Autodesk Fusion 360 part; units mm, degrees
(part 7 of 7)
  spline S2021 degree 3 poles (-41.0081, 27.0862) (-40.9963, 27.0636) (-41.0844, 27.0271) (-41.1005, 27.0604) knots 0 0 0 0 1 1 1 1
  spline S2022 degree 3 poles (-41.1005, 27.0604) (-41.1284, 27.1281) (-41.1295, 27.1399) (-41.1349, 27.1904) knots 0 0 0 0 1 1 1 1
  spline S2023 degree 3 poles (-38.245, 28.2123) (-38.2557, 28.2779) (-38.1913, 28.3445) (-38.1558, 28.251) knots 0 0 0 0 1 1 1 1
  spline S2024 degree 3 poles (-38.1558, 28.251) (-38.1258, 28.1715) (-38.129, 28.1296) (-38.1182, 28.107) knots 0 0 0 0 1 1 1 1
  spline S2025 degree 3 poles (-38.1182, 28.107) (-38.1064, 28.0845) (-38.1945, 28.049) (-38.2106, 28.0823) knots 0 0 0 0 1 1 1 1
  spline S2026 degree 3 poles (-38.2106, 28.0823) (-38.2386, 28.1489) (-38.2396, 28.1618) (-38.245, 28.2123) knots 0 0 0 0 1 1 1 1
  spline S2027 degree 3 poles (-40.9179, 27.2764) (-40.9318, 27.3473) (-40.8609, 27.4236) (-40.8233, 27.3258) knots 0 0 0 0 1 1 1 1
  spline S2028 degree 3 poles (-40.8233, 27.3258) (-40.789, 27.2398) (-40.7954, 27.199) (-40.7804, 27.1689) knots 0 0 0 0 1 1 1 1
  spline S2029 degree 3 poles (-40.7804, 27.1689) (-40.7664, 27.1388) (-40.8609, 27.098) (-40.8803, 27.1377) knots 0 0 0 0 1 1 1 1
  spline S2030 degree 3 poles (-40.8803, 27.1377) (-40.9082, 27.2033) (-40.9104, 27.2259) (-40.9179, 27.2764) knots 0 0 0 0 1 1 1 1
  spline S2031 degree 3 poles (-38.4889, 28.1468) (-38.5039, 28.2177) (-38.4341, 28.294) (-38.3954, 28.1962) knots 0 0 0 0 1 1 1 1
  spline S2032 degree 3 poles (-38.3954, 28.1962) (-38.361, 28.1103) (-38.3685, 28.0705) (-38.3535, 28.0404) knots 0 0 0 0 1 1 1 1
  spline S2033 degree 3 poles (-38.3535, 28.0404) (-38.3385, 28.0103) (-38.4341, 27.9695) (-38.4523, 28.0082) knots 0 0 0 0 1 1 1 1
  spline S2034 degree 3 poles (-38.4523, 28.0082) (-38.4813, 28.0748) (-38.4824, 28.0963) (-38.4889, 28.1468) knots 0 0 0 0 1 1 1 1
  spline S2035 degree 3 poles (-40.6998, 27.3613) (-40.7181, 27.4386) (-40.6418, 27.5224) (-40.601, 27.4214) knots 0 0 0 0 1 1 1 1
  spline S2036 degree 3 poles (-40.601, 27.4214) (-40.5644, 27.329) (-40.572, 27.2903) (-40.5537, 27.2527) knots 0 0 0 0 1 1 1 1
  spline S2037 degree 3 poles (-40.5537, 27.2527) (-40.5354, 27.2151) (-40.6386, 27.1689) (-40.66, 27.214) knots 0 0 0 0 1 1 1 1
  spline S2038 degree 3 poles (-40.66, 27.214) (-40.6901, 27.2807) (-40.6901, 27.3118) (-40.6998, 27.3613) knots 0 0 0 0 1 1 1 1
  spline S2039 degree 3 poles (-38.737, 28.0307) (-38.7553, 28.107) (-38.679, 28.1919) (-38.6382, 28.0909) knots 0 0 0 0 1 1 1 1
  spline S2040 degree 3 poles (-38.6382, 28.0909) (-38.6006, 27.9985) (-38.6092, 27.9587) (-38.5909, 27.9211) knots 0 0 0 0 1 1 1 1
  spline S2041 degree 3 poles (-38.5909, 27.9211) (-38.5727, 27.8846) (-38.6758, 27.8373) (-38.6973, 27.8824) knots 0 0 0 0 1 1 1 1
  spline S2042 degree 3 poles (-38.6973, 27.8824) (-38.7263, 27.9491) (-38.7274, 27.9802) (-38.737, 28.0307) knots 0 0 0 0 1 1 1 1
  spline S2043 degree 3 poles (-40.4828, 27.4472) (-40.5043, 27.5289) (-40.4216, 27.6224) (-40.3786, 27.5171) knots 0 0 0 0 1 1 1 1
  spline S2044 degree 3 poles (-40.3786, 27.5171) (-40.3388, 27.4193) (-40.3496, 27.3817) (-40.3259, 27.3366) knots 0 0 0 0 1 1 1 1
  spline S2045 degree 3 poles (-40.3259, 27.3366) (-40.3044, 27.2914) (-40.4151, 27.2398) (-40.4398, 27.2903) knots 0 0 0 0 1 1 1 1
  spline S2046 degree 3 poles (-40.4398, 27.2903) (-40.471, 27.357) (-40.471, 27.3967) (-40.4828, 27.4472) knots 0 0 0 0 1 1 1 1
  spline S2047 degree 3 poles (-39.0443, 27.9534) (-39.0658, 28.034) (-38.982, 28.1285) (-38.9401, 28.0232) knots 0 0 0 0 1 1 1 1
  spline S2048 degree 3 poles (-38.9401, 28.0232) (-38.8993, 27.9243) (-38.91, 27.8867) (-38.8874, 27.8416) knots 0 0 0 0 1 1 1 1
  spline S2049 degree 3 poles (-38.8874, 27.8416) (-38.8659, 27.7976) (-38.9777, 27.7449) (-39.0013, 27.7954) knots 0 0 0 0 1 1 1 1
  spline S2050 degree 3 poles (-39.0013, 27.7954) (-39.0314, 27.8631) (-39.0325, 27.9029) (-39.0443, 27.9534) knots 0 0 0 0 1 1 1 1
  spline S2051 degree 3 poles (-39.2119, 28.5068) (-39.2334, 28.5884) (-39.1517, 28.6819) (-39.1087, 28.5777) knots 0 0 0 0 1 1 1 1
  spline S2052 degree 3 poles (-39.1087, 28.5777) (-39.0668, 28.4788) (-39.0776, 28.4412) (-39.0561, 28.3961) knots 0 0 0 0 1 1 1 1
  spline S2053 degree 3 poles (-39.0561, 28.3961) (-39.0335, 28.351) (-39.1453, 28.2994) (-39.1689, 28.3499) knots 0 0 0 0 1 1 1 1
  spline S2054 degree 3 poles (-39.1689, 28.3499) (-39.2001, 28.4176) (-39.2011, 28.4573) (-39.2119, 28.5068) knots 0 0 0 0 1 1 1 1
  spline S2055 degree 3 poles (-39.6319, 28.9774) (-39.6523, 29.058) (-39.5707, 29.1526) (-39.5277, 29.0473) knots 0 0 0 0 1 1 1 1
  spline S2056 degree 3 poles (-39.5277, 29.0473) (-39.4869, 28.9484) (-39.4976, 28.9108) (-39.4751, 28.8657) knots 0 0 0 0 1 1 1 1
  spline S2057 degree 3 poles (-39.4751, 28.8657) (-39.4536, 28.8216) (-39.5642, 28.769) (-39.589, 28.8206) knots 0 0 0 0 1 1 1 1
  spline S2058 degree 3 poles (-39.589, 28.8206) (-39.619, 28.8872) (-39.6201, 28.9269) (-39.6319, 28.9774) knots 0 0 0 0 1 1 1 1
  spline S2059 degree 3 poles (-40.2325, 27.5332) (-40.2561, 27.6192) (-40.1691, 27.7223) (-40.1229, 27.6127) knots 0 0 0 0 1 1 1 1
  spline S2060 degree 3 poles (-40.1229, 27.6127) (-40.0799, 27.5085) (-40.0928, 27.4719) (-40.066, 27.4193) knots 0 0 0 0 1 1 1 1
  spline S2061 degree 3 poles (-40.066, 27.4193) (-40.0402, 27.3677) (-40.1583, 27.3108) (-40.1863, 27.3666) knots 0 0 0 0 1 1 1 1
  spline S2062 degree 3 poles (-40.1863, 27.3666) (-40.2185, 27.4343) (-40.2185, 27.4827) (-40.2325, 27.5332) knots 0 0 0 0 1 1 1 1
  spline S2063 degree 3 poles (-39.2409, 27.8685) (-39.2656, 27.9544) (-39.1775, 28.0576) (-39.1324, 27.948) knots 0 0 0 0 1 1 1 1
  spline S2064 degree 3 poles (-39.1324, 27.948) (-39.0883, 27.8438) (-39.1012, 27.8072) (-39.0744, 27.7546) knots 0 0 0 0 1 1 1 1
  spline S2065 degree 3 poles (-39.0744, 27.7546) (-39.0486, 27.703) (-39.1678, 27.646) (-39.1958, 27.7008) knots 0 0 0 0 1 1 1 1
  spline S2066 degree 3 poles (-39.1958, 27.7008) (-39.2269, 27.7685) (-39.2269, 27.818) (-39.2409, 27.8685) knots 0 0 0 0 1 1 1 1
  spline S2067 degree 3 poles (-39.1163, 27.3097) (-39.1421, 27.3967) (-39.054, 27.4988) (-39.0088, 27.3903) knots 0 0 0 0 1 1 1 1
  spline S2068 degree 3 poles (-39.0088, 27.3903) (-38.9648, 27.285) (-38.9777, 27.2484) (-38.9508, 27.1968) knots 0 0 0 0 1 1 1 1
  spline S2069 degree 3 poles (-38.9508, 27.1968) (-38.925, 27.1442) (-39.0432, 27.0872) (-39.0711, 27.1431) knots 0 0 0 0 1 1 1 1
  spline S2070 degree 3 poles (-39.0711, 27.1431) (-39.1034, 27.2097) (-39.1034, 27.2592) (-39.1163, 27.3097) knots 0 0 0 0 1 1 1 1
  spline S2071 degree 3 poles (-40.0133, 27.6192) (-40.0434, 27.7105) (-39.9489, 27.8223) (-39.9016, 27.7094) knots 0 0 0 0 1 1 1 1
  spline S2072 degree 3 poles (-39.9016, 27.7094) (-39.8543, 27.5977) (-39.8693, 27.5622) (-39.8393, 27.5031) knots 0 0 0 0 1 1 1 1
  spline S2073 degree 3 poles (-39.8393, 27.5031) (-39.8092, 27.444) (-39.936, 27.3817) (-39.966, 27.4429) knots 0 0 0 0 1 1 1 1
  spline S2074 degree 3 poles (-39.966, 27.4429) (-39.9993, 27.5106) (-39.9993, 27.5687) (-40.0133, 27.6192) knots 0 0 0 0 1 1 1 1
  spline S2075 degree 3 poles (-39.5234, 27.7814) (-39.5524, 27.8728) (-39.459, 27.9856) (-39.4106, 27.8728) knots 0 0 0 0 1 1 1 1
  spline S2076 degree 3 poles (-39.4106, 27.8728) (-39.3634, 27.761) (-39.3784, 27.7256) (-39.3483, 27.6664) knots 0 0 0 0 1 1 1 1
  spline S2077 degree 3 poles (-39.3483, 27.6664) (-39.3182, 27.6063) (-39.445, 27.544) (-39.4751, 27.6063) knots 0 0 0 0 1 1 1 1
  spline S2078 degree 3 poles (-39.4751, 27.6063) (-39.5084, 27.6729) (-39.5084, 27.7309) (-39.5234, 27.7814) knots 0 0 0 0 1 1 1 1
  spline S2079 degree 3 poles (-39.7963, 27.7041) (-39.8296, 27.8008) (-39.7297, 27.9222) (-39.6792, 27.8051) knots 0 0 0 0 1 1 1 1
  spline S2080 degree 3 poles (-39.6792, 27.8051) (-39.6287, 27.6879) (-39.6459, 27.6536) (-39.6115, 27.5869) knots 0 0 0 0 1 1 1 1
  spline S2081 degree 3 poles (-39.6115, 27.5869) (-39.5782, 27.5192) (-39.7125, 27.4526) (-39.7458, 27.5192) knots 0 0 0 0 1 1 1 1
  spline S2082 degree 3 poles (-39.7458, 27.5192) (-39.7802, 27.5869) (-39.7802, 27.6535) (-39.7963, 27.7041) knots 0 0 0 0 1 1 1 1
  spline S2083 degree 3 poles (-38.0409, 26.9218) (-37.6047, 26.6145) (-37.1127, 26.1287) (-36.6357, 25.6559) knots 0 0 0 0 1 1 1 1
  line L728 (-36.6357, 25.6559) -> (-36.554, 25.5753)
  spline S2084 degree 3 poles (-36.554, 25.5753) (-36.4906, 25.7516) (-36.3563, 26.0696) (-36.2382, 26.0847) knots 0 0 0 0 1 1 1 1
  spline S2085 degree 3 poles (-36.2382, 26.0847) (-36.0953, 26.1008) (-35.8267, 26.0847) (-35.7171, 25.9665) knots 0 0 0 0 1 1 1 1
  spline S2086 degree 3 poles (-35.7171, 25.9665) (-35.6086, 25.8493) (-35.4571, 25.6387) (-35.4743, 25.513) knots 0 0 0 0 1 1 1 1
  spline S2087 degree 3 poles (-35.4743, 25.513) (-35.4905, 25.3873) (-35.5409, 25.3368) (-35.6505, 25.3368) knots 0 0 0 0 1 1 1 1
  spline S2088 degree 3 poles (-35.6505, 25.3368) (-35.759, 25.3368) (-35.802, 25.4464) (-35.8095, 25.5388) knots 0 0 0 0 1 1 1 1
  spline S2089 degree 3 poles (-35.8095, 25.5388) (-35.8181, 25.6312) (-35.9019, 25.6978) (-35.9696, 25.6978) knots 0 0 0 0 1 1 1 1
  spline S2090 degree 3 poles (-35.9696, 25.6978) (-36.0362, 25.6978) (-36.1039, 25.614) (-36.1877, 25.5388) knots 0 0 0 0 1 1 1 1
  spline S2091 degree 3 poles (-36.1877, 25.5388) (-36.2437, 25.4825) (-36.3116, 25.4396) (-36.3864, 25.4131) knots 0 0 0 0 1 1 1 1
  line L729 (-36.3864, 25.4131) -> (-36.1737, 25.2035)
  spline S2092 degree 3 poles (-36.1737, 25.2035) (-35.7923, 24.8382) (-35.4475, 24.922) (-35.2691, 25.1057) knots 0 0 0 0 1 1 1 1
  spline S2093 degree 3 poles (-35.2691, 25.1057) (-35.1155, 25.2626) (-35.0489, 25.527) (-35.2294, 25.7064) knots 0 0 0 0 1 1 1 1
  spline S2094 degree 3 poles (-35.2294, 25.7064) (-35.4894, 25.9675) (-35.9492, 26.4576) (-36.3059, 26.8423) knots 0 0 0 0 1 1 1 1
  spline S2095 degree 3 poles (-36.3059, 26.8423) (-36.5895, 26.9916) (-36.7377, 27.2248) (-36.799, 27.3495) knots 0 0 0 0 1 1 1 1
  spline S2096 degree 3 poles (-36.799, 27.3495) (-37.2096, 27.1975) (-37.6237, 27.0548) (-38.0409, 26.9218) knots 0 0 0 0 1 1 1 1
  spline S2097 degree 3 poles (-36.1125, 26.1599) (-36.1888, 26.147) (-35.9363, 26.3103) (-35.9363, 26.2265) knots 0 0 0 0 1 1 1 1
  spline S2098 degree 3 poles (-35.9363, 26.2265) (-35.9363, 26.1427) (-36.0115, 26.176) (-36.1125, 26.1599) knots 0 0 0 0 1 1 1 1
  spline S2099 degree 2 poles (-37.8164, 26.9239) (-37.1277, 27.1926) (-37.0267, 27.2087) knots 0 0 0 1 1 1
  spline S2100 degree 3 poles (-37.0267, 27.2087) (-36.9257, 27.2259) (-36.8839, 27.1421) (-37.0106, 27.1087) knots 0 0 0 0 1 1 1 1
  spline S2101 degree 3 poles (-37.0106, 27.1087) (-37.1363, 27.0744) (-37.9335, 26.7219) (-37.8164, 26.9239) knots 0 0 0 0 1 1 1 1
  spline S2102 degree 3 poles (-37.5811, 26.8057) (-37.4575, 26.8551) (-37.0944, 26.9905) (-36.9762, 27.0077) knots 0 0 0 0 1 1 1 1
  spline S2103 degree 3 poles (-36.9762, 27.0077) (-36.8592, 27.0249) (-36.7249, 26.94) (-36.8505, 26.882) knots 0 0 0 0 1 1 1 1
  spline S2104 degree 3 poles (-36.8505, 26.882) (-36.9762, 26.8229) (-37.3791, 26.6553) (-37.4618, 26.6553) knots 0 0 0 0 1 1 1 1
  spline S2105 degree 3 poles (-37.4618, 26.6553) (-37.5478, 26.6553) (-37.6649, 26.7724) (-37.5811, 26.8057) knots 0 0 0 0 1 1 1 1
  spline S2106 degree 3 poles (-37.2362, 26.6134) (-37.1449, 26.6692) (-36.8334, 26.7649) (-36.7335, 26.7907) knots 0 0 0 0 1 1 1 1
  spline S2107 degree 3 poles (-36.7335, 26.7907) (-36.6325, 26.8154) (-36.322, 26.7563) (-36.5401, 26.6897) knots 0 0 0 0 1 1 1 1
  spline S2108 degree 3 poles (-36.5401, 26.6897) (-36.7412, 26.6215) (-36.9375, 26.5401) (-37.1277, 26.4457) knots 0 0 0 0 1 1 1 1
  spline S2109 degree 3 poles (-37.1277, 26.4457) (-37.1943, 26.4113) (-37.4049, 26.5124) (-37.2362, 26.6134) knots 0 0 0 0 1 1 1 1
  spline S2110 degree 3 poles (-36.9677, 26.3866) (-36.8344, 26.4973) (-36.5487, 26.579) (-36.4649, 26.6123) knots 0 0 0 0 1 1 1 1
  spline S2111 degree 3 poles (-36.4649, 26.6123) (-36.3811, 26.6456) (-36.2715, 26.5618) (-36.3886, 26.4952) knots 0 0 0 0 1 1 1 1
  spline S2112 degree 3 poles (-36.3886, 26.4952) (-36.5068, 26.4285) (-36.6658, 26.378) (-36.7839, 26.3028) knots 0 0 0 0 1 1 1 1
  spline S2113 degree 3 poles (-36.7839, 26.3028) (-36.901, 26.2265) (-37.0686, 26.3028) (-36.9677, 26.3866) knots 0 0 0 0 1 1 1 1
  spline S2114 degree 3 poles (-36.683, 26.1599) (-36.6271, 26.2845) (-36.4305, 26.3694) (-36.3392, 26.378) knots 0 0 0 0 1 1 1 1
  spline S2115 degree 3 poles (-36.3392, 26.378) (-36.2468, 26.3866) (-36.0781, 26.4199) (-36.1544, 26.3275) knots 0 0 0 0 1 1 1 1
  spline S2116 degree 3 poles (-36.1544, 26.3275) (-36.2296, 26.2351) (-36.4144, 26.0847) (-36.5326, 26.0589) knots 0 0 0 0 1 1 1 1
  spline S2117 degree 3 poles (-36.5326, 26.0589) (-36.6497, 26.0342) (-36.7163, 26.0847) (-36.683, 26.1599) knots 0 0 0 0 1 1 1 1
  line L730 (-33.0754, 24.504) -> (-33.4256, 24.5566)
  spline S2118 degree 3 poles (-33.4256, 24.5566) (-33.6254, 24.5878) (-33.8854, 24.6222) (-34.1057, 24.6985) knots 0 0 0 0 1 1 1 1
  spline S2119 degree 3 poles (-34.1057, 24.6985) (-33.8858, 24.621) (-33.6597, 24.5624) (-33.4299, 24.5233) knots 0 0 0 0 1 1 1 1
  spline S2120 degree 3 poles (-33.4299, 24.5233) (-33.2279, 24.4922) (-33.0775, 24.504) (-33.0754, 24.504) knots 0 0 0 0 1 1 1 1
  spline S2121 degree 3 poles (-33.5245, 24.2804) (-33.5245, 24.2794) (-33.5835, 24.2848) (-33.6716, 24.288) knots 0 0 0 0 1 1 1 1
  spline S2122 degree 3 poles (-33.6716, 24.288) (-33.7597, 24.2901) (-33.8854, 24.2858) (-34.0154, 24.3181) knots 0 0 0 0 1 1 1 1
  spline S2123 degree 3 poles (-34.0154, 24.3181) (-33.9031, 24.286) (-33.788, 24.2644) (-33.6716, 24.2536) knots 0 0 0 0 1 1 1 1
  spline S2124 degree 3 poles (-33.6716, 24.2536) (-33.6211, 24.2506) (-33.5706, 24.2598) (-33.5245, 24.2804) knots 0 0 0 0 1 1 1 1
  line L731 (-34.53, 23.8098) -> (-34.8469, 23.8807)
  spline S2125 degree 3 poles (-34.8469, 23.8807) (-35.022, 23.9194) (-35.2391, 23.9602) (-35.3819, 24.0258) knots 0 0 0 0 1 1 1 1
  spline S2126 degree 3 poles (-35.3819, 24.0258) (-35.2125, 23.95) (-35.0362, 23.8906) (-34.8555, 23.8485) knots 0 0 0 0 1 1 1 1
  spline S2127 degree 3 poles (-34.8555, 23.8485) (-34.6783, 23.8098) (-34.5332, 23.8109) (-34.53, 23.8098) knots 0 0 0 0 1 1 1 1
  spline S2128 degree 3 poles (-35.1348, 23.6529) (-35.179, 23.6655) (-35.223, 23.6784) (-35.267, 23.6916) knots 0 0 0 0 1 1 1 1
  spline S2129 degree 3 poles (-35.267, 23.6916) (-35.3443, 23.7141) (-35.4518, 23.7378) (-35.5377, 23.8033) knots 0 0 0 0 1 1 1 1
  spline S2130 degree 3 poles (-35.5377, 23.8033) (-35.4603, 23.7409) (-35.3727, 23.6922) (-35.2788, 23.6593) knots 0 0 0 0 1 1 1 1
  spline S2131 degree 3 poles (-35.2788, 23.6593) (-35.1993, 23.6368) (-35.1391, 23.654) (-35.1348, 23.6529) knots 0 0 0 0 1 1 1 1
  line L732 (-35.5839, 23.5637) -> (-35.6881, 23.5766)
  spline S2132 degree 3 poles (-35.6881, 23.5766) (-35.7483, 23.5852) (-35.8331, 23.5938) (-35.8965, 23.6464) knots 0 0 0 0 1 1 1 1
  spline S2133 degree 3 poles (-35.8965, 23.6464) (-35.84, 23.5947) (-35.7706, 23.5591) (-35.6956, 23.5433) knots 0 0 0 0 1 1 1 1
  spline S2134 degree 3 poles (-35.6956, 23.5433) (-35.6301, 23.5347) (-35.5871, 23.5626) (-35.5839, 23.5637) knots 0 0 0 0 1 1 1 1
  spline S2135 degree 3 poles (-37.0149, 23.8259) (-36.959, 23.7571) (-36.8129, 23.6636) (-36.6657, 23.5959) knots 0 0 0 0 1 1 1 1
  spline S2136 degree 3 poles (-36.6657, 23.5959) (-36.5186, 23.5293) (-36.3757, 23.5003) (-36.3638, 23.496) knots 0 0 0 0 1 1 1 1
  spline S2137 degree 3 poles (-36.3638, 23.496) (-36.3671, 23.496) (-36.4971, 23.5562) (-36.6432, 23.6228) knots 0 0 0 0 1 1 1 1
  spline S2138 degree 3 poles (-36.6432, 23.6228) (-36.7893, 23.6894) (-36.9622, 23.7614) (-37.0149, 23.8259) knots 0 0 0 0 1 1 1 1
  spline S2139 degree 3 poles (-37.2383, 23.6389) (-37.3135, 23.6873) (-37.4092, 23.7378) (-37.4414, 23.7808) knots 0 0 0 0 1 1 1 1
  spline S2140 degree 3 poles (-37.4414, 23.7808) (-37.3907, 23.7162) (-37.3301, 23.66) (-37.262, 23.6142) knots 0 0 0 0 1 1 1 1
  spline S2141 degree 3 poles (-37.262, 23.6142) (-37.1868, 23.5626) (-37.1073, 23.5433) (-37.1008, 23.5401) knots 0 0 0 0 1 1 1 1
  spline S2142 degree 3 poles (-37.1008, 23.5401) (-37.103, 23.5411) (-37.1642, 23.5895) (-37.2383, 23.6389) knots 0 0 0 0 1 1 1 1
  spline S2143 degree 3 poles (-37.9549, 23.7582) (-37.9512, 23.7313) (-37.9417, 23.7056) (-37.927, 23.6828) knots 0 0 0 0 1 1 1 1
  spline S2144 degree 3 poles (-37.927, 23.6828) (-37.9124, 23.6599) (-37.8929, 23.6406) (-37.87, 23.626) knots 0 0 0 0 1 1 1 1
  spline S2145 degree 3 poles (-37.87, 23.626) (-37.826, 23.5992) (-37.7776, 23.6078) (-37.7744, 23.6067) knots 0 0 0 0 1 1 1 1
  spline S2146 degree 3 poles (-37.7744, 23.6067) (-37.7989, 23.6217) (-37.8236, 23.6364) (-37.8485, 23.6507) knots 0 0 0 0 1 1 1 1
  spline S2147 degree 3 poles (-37.8485, 23.6507) (-37.8872, 23.6754) (-37.9463, 23.7077) (-37.9549, 23.7582) knots 0 0 0 0 1 1 1 1
  spline S2148 degree 3 poles (-38.2804, 23.6185) (-38.2106, 23.5734) (-38.1364, 23.5658) (-38.1311, 23.5626) knots 0 0 0 0 1 1 1 1
  line L733 (-38.1311, 23.5626) -> (-38.2579, 23.6443)
  spline S2149 degree 3 poles (-38.2579, 23.6443) (-38.3255, 23.6873) (-38.4158, 23.7389) (-38.448, 23.8033) knots 0 0 0 0 1 1 1 1
  spline S2150 degree 3 poles (-38.448, 23.8033) (-38.4089, 23.7284) (-38.3512, 23.6647) (-38.2804, 23.6185) knots 0 0 0 0 1 1 1 1
  line L734 (-47.4679, 29.1537) -> (-47.2176, 29.1935)
  line L735 (-47.2176, 29.1935) -> (-46.9758, 29.2655)
  line L736 (-46.9758, 29.2655) -> (-47.2251, 29.2268)
  line L737 (-47.2251, 29.2268) -> (-47.4679, 29.1537)
  line L738 (-47.4109, 32.6731) -> (-47.4131, 32.6623)
  line L739 (-47.4131, 32.6623) -> (-47.2713, 32.6075)
  line L740 (-47.2713, 32.6075) -> (-47.1101, 32.572)
  line L741 (-47.1101, 32.572) -> (-47.1069, 32.5806)
  line L742 (-47.1069, 32.5806) -> (-47.2605, 32.6397)
  line L743 (-47.2605, 32.6397) -> (-47.4109, 32.6731)
  spline S2151 degree 3 poles (-47.4786, 32.3797) (-47.4788, 32.376) (-47.4796, 32.3724) (-47.4808, 32.3689) knots 0 0 0 0 1 1 1 1
  line L744 (-47.4808, 32.3689) -> (-47.3272, 32.3055)
  line L745 (-47.3272, 32.3055) -> (-47.1982, 32.2722)
  spline S2152 degree 3 poles (-47.1982, 32.2722) (-47.1966, 32.2772) (-47.1952, 32.2822) (-47.1939, 32.2873) knots 0 0 0 0 1 1 1 1
  line L746 (-47.1939, 32.2873) -> (-47.3164, 32.3378)
  line L747 (-47.3164, 32.3378) -> (-47.4786, 32.3797)
  line L748 (-47.5377, 32.0745) -> (-47.5399, 32.0648)
  line L749 (-47.5399, 32.0648) -> (-47.4045, 32.0143)
  line L750 (-47.4045, 32.0143) -> (-47.2605, 31.9864)
  line L751 (-47.2605, 31.9864) -> (-47.2584, 31.9971)
  line L752 (-47.2584, 31.9971) -> (-47.3959, 32.0455)
  line L753 (-47.3959, 32.0455) -> (-47.5377, 32.0745)
  line L754 (-47.3357, 32.9632) -> (-47.3379, 32.9546)
  line L755 (-47.3379, 32.9546) -> (-47.1714, 32.8761)
  line L756 (-47.1714, 32.8761) -> (-47.007, 32.8267)
  line L757 (-47.007, 32.8267) -> (-47.0027, 32.8364)
  line L758 (-47.0027, 32.8364) -> (-47.1596, 32.9084)
  line L759 (-47.1596, 32.9084) -> (-47.3357, 32.9632)
  line L760 (-47.628, 31.4663) -> (-47.629, 31.4545)
  line L761 (-47.629, 31.4545) -> (-47.4797, 31.4426)
  line L762 (-47.4797, 31.4426) -> (-47.2938, 31.4587)
  line L763 (-47.2938, 31.4587) -> (-47.2949, 31.463)
  line L764 (-47.2949, 31.463) -> (-47.4797, 31.477)
  line L765 (-47.4797, 31.477) -> (-47.628, 31.4663)
  line L766 (-47.5947, 31.7199) -> (-47.5968, 31.7059)
  line L767 (-47.5968, 31.7059) -> (-47.4808, 31.678)
  line L768 (-47.4808, 31.678) -> (-47.3153, 31.6661)
  line L769 (-47.3153, 31.6661) -> (-47.3153, 31.6715)
  line L770 (-47.3153, 31.6715) -> (-47.4765, 31.7113)
  line L771 (-47.4765, 31.7113) -> (-47.5947, 31.7199)
  line L772 (-47.6559, 31.1976) -> (-47.658, 31.1815)
  line L773 (-47.658, 31.1815) -> (-47.5098, 31.1976)
  line L774 (-47.5098, 31.1976) -> (-47.2638, 31.2546)
  line L775 (-47.2638, 31.2546) -> (-47.5152, 31.2299)
  line L776 (-47.5152, 31.2299) -> (-47.6559, 31.1976)
  line L777 (-47.6795, 30.8774) -> (-47.6806, 30.8688)
  line L778 (-47.6806, 30.8688) -> (-47.4528, 30.9053)
  line L779 (-47.4528, 30.9053) -> (-47.2122, 30.973)
  line L780 (-47.2122, 30.973) -> (-47.2143, 30.9795)
  line L781 (-47.2143, 30.9795) -> (-47.4604, 30.9397)
  line L782 (-47.4604, 30.9397) -> (-47.6795, 30.8774)
  line L783 (-47.6903, 30.6625) -> (-47.6903, 30.6517)
  line L784 (-47.6903, 30.6517) -> (-47.4528, 30.6947)
  line L785 (-47.4528, 30.6947) -> (-47.1714, 30.771)
  line L786 (-47.1714, 30.771) -> (-47.1725, 30.7764)
  line L787 (-47.1725, 30.7764) -> (-47.4604, 30.7259)
  line L788 (-47.4604, 30.7259) -> (-47.6903, 30.6625)
  line L789 (-47.6967, 30.3444) -> (-47.6967, 30.3369)
  line L790 (-47.6967, 30.3369) -> (-47.3959, 30.4024)
  line L791 (-47.3959, 30.4024) -> (-47.1058, 30.4927)
  line L792 (-47.1058, 30.4927) -> (-47.108, 30.5002)
  line L793 (-47.108, 30.5002) -> (-47.4045, 30.4347)
  line L794 (-47.4045, 30.4347) -> (-47.6967, 30.3444)
  line L795 (-47.2208, 30.2058) -> (-47.484, 30.1434)
  line L796 (-47.484, 30.1434) -> (-47.6935, 30.065)
  line L797 (-47.6935, 30.065) -> (-47.6935, 30.0596)
  line L798 (-47.6935, 30.0596) -> (-47.4743, 30.1112)
  line L799 (-47.4743, 30.1112) -> (-47.2208, 30.2058)
  line L800 (-47.1316, 29.9833) -> (-47.4496, 29.9199)
  line L801 (-47.4496, 29.9199) -> (-47.686, 29.8479)
  line L802 (-47.686, 29.8479) -> (-47.686, 29.8393)
  line L803 (-47.686, 29.8393) -> (-47.441, 29.8877)
  line L804 (-47.441, 29.8877) -> (-47.1316, 29.9833)
  line L805 (-47.1767, 29.7351) -> (-47.4733, 29.6502)
  line L806 (-47.4733, 29.6502) -> (-47.6699, 29.5707)
  line L807 (-47.6699, 29.5707) -> (-47.6688, 29.5599)
  line L808 (-47.6688, 29.5599) -> (-47.4625, 29.619)
  line L809 (-47.4625, 29.619) -> (-47.1767, 29.7351)
  line L810 (-47.1101, 28.7508) -> (-47.3615, 28.6659)
  line L811 (-47.3615, 28.6659) -> (-47.5474, 28.5756)
  line L812 (-47.5474, 28.5756) -> (-47.5463, 28.5681)
  line L813 (-47.5463, 28.5681) -> (-47.3497, 28.6347)
  line L814 (-47.3497, 28.6347) -> (-47.1101, 28.7508)
  spline S2153 degree 3 poles (-47.3336, 28.3929) (-47.325, 28.3951) (-47.2186, 28.4069) (-47.094, 28.4488) knots 0 0 0 0 1 1 1 1
  spline S2154 degree 3 poles (-47.094, 28.4488) (-46.9694, 28.4907) (-46.8298, 28.5606) (-46.7288, 28.6164) knots 0 0 0 0 1 1 1 1
  spline S2155 degree 3 poles (-46.7288, 28.6164) (-46.8276, 28.5616) (-46.9855, 28.5208) (-47.1101, 28.4789) knots 0 0 0 0 1 1 1 1
  spline S2156 degree 3 poles (-47.1101, 28.4789) (-47.2348, 28.437) (-47.3314, 28.3929) (-47.3336, 28.3929) knots 0 0 0 0 1 1 1 1
  spline S2157 degree 3 poles (-47.2659, 28.1243) (-47.2573, 28.1254) (-47.1338, 28.1318) (-47.0006, 28.1683) knots 0 0 0 0 1 1 1 1
  spline S2158 degree 3 poles (-47.0006, 28.1683) (-46.8793, 28.2) (-46.7647, 28.2531) (-46.6622, 28.3252) knots 0 0 0 0 1 1 1 1
  spline S2159 degree 3 poles (-46.6622, 28.3252) (-46.7266, 28.2715) (-46.8856, 28.235) (-47.0178, 28.1995) knots 0 0 0 0 1 1 1 1
  spline S2160 degree 3 poles (-47.0178, 28.1995) (-47.1499, 28.164) (-47.2638, 28.1243) (-47.2659, 28.1243) knots 0 0 0 0 1 1 1 1
  spline S2161 degree 3 poles (-47.2208, 27.8556) (-47.2122, 27.8567) (-47.0897, 27.8632) (-46.9587, 27.9008) knots 0 0 0 0 1 1 1 1
  spline S2162 degree 3 poles (-46.9587, 27.9008) (-46.8475, 27.9283) (-46.743, 27.978) (-46.6514, 28.0469) knots 0 0 0 0 1 1 1 1
  spline S2163 degree 3 poles (-46.6514, 28.0469) (-46.7126, 27.9985) (-46.8555, 27.9642) (-46.9769, 27.9309) knots 0 0 0 0 1 1 1 1
  spline S2164 degree 3 poles (-46.9769, 27.9309) (-47.1058, 27.8954) (-47.2186, 27.8556) (-47.2208, 27.8556) knots 0 0 0 0 1 1 1 1
  line L815 (-47.0425, 27.631) -> (-46.7674, 27.7396)
  line L816 (-46.7674, 27.7396) -> (-46.5053, 27.8771)
  line L817 (-46.5053, 27.8771) -> (-46.7803, 27.7697)
  line L818 (-46.7803, 27.7697) -> (-47.0425, 27.631)
  line L819 (-47.065, 27.3183) -> (-46.7664, 27.4602)
  line L820 (-46.7664, 27.4602) -> (-46.4827, 27.631)
  line L821 (-46.4827, 27.631) -> (-46.7814, 27.4903)
  line L822 (-46.7814, 27.4903) -> (-47.065, 27.3183)
  line L823 (-46.9758, 27.0937) -> (-46.5655, 27.2463)
  line L824 (-46.5655, 27.2463) -> (-46.1701, 27.4301)
  line L825 (-46.1701, 27.4301) -> (-46.5794, 27.2775)
  line L826 (-46.5794, 27.2775) -> (-46.9758, 27.0937)
  line L827 (-46.8856, 26.8251) -> (-46.5537, 26.9669)
  line L828 (-46.5537, 26.9669) -> (-46.2367, 27.1389)
  line L829 (-46.2367, 27.1389) -> (-46.5687, 26.9981)
  line L830 (-46.5687, 26.9981) -> (-46.8856, 26.8251)
  line L831 (-46.7073, 26.5124) -> (-46.3732, 26.6994)
  line L832 (-46.3732, 26.6994) -> (-46.0573, 26.9154)
  line L833 (-46.0573, 26.9154) -> (-46.3914, 26.7284)
  line L834 (-46.3914, 26.7284) -> (-46.7073, 26.5124)
  line L835 (-46.5945, 26.2878) -> (-46.1841, 26.5199)
  line L836 (-46.1841, 26.5199) -> (-45.7887, 26.781)
  line L837 (-45.7887, 26.781) -> (-46.2002, 26.5489)
  line L838 (-46.2002, 26.5489) -> (-46.5945, 26.2878)
  line L839 (-46.5494, 26.0417) -> (-46.0272, 26.3297)
  line L840 (-46.0272, 26.3297) -> (-45.5202, 26.6467)
  line L841 (-45.5202, 26.6467) -> (-46.0444, 26.3598)
  line L842 (-46.0444, 26.3598) -> (-46.5494, 26.0417)
  line L843 (-46.4387, 25.7731) -> (-46.0262, 26.0396)
  line L844 (-46.0262, 26.0396) -> (-45.633, 26.3329)
  line L845 (-45.633, 26.3329) -> (-46.0455, 26.0664)
  line L846 (-46.0455, 26.0664) -> (-46.4387, 25.7731)
  line L847 (-46.1024, 25.7064) -> (-45.7232, 25.9493)
  line L848 (-45.7232, 25.9493) -> (-45.3644, 26.2212)
  line L849 (-45.3644, 26.2212) -> (-45.7426, 25.9772)
  line L850 (-45.7426, 25.9772) -> (-46.1024, 25.7064)
  line L851 (-46.125, 25.3701) -> (-45.6222, 25.715)
  line L852 (-45.6222, 25.715) -> (-45.1399, 26.0868)
  line L853 (-45.1399, 26.0868) -> (-45.6426, 25.7419)
  line L854 (-45.6426, 25.7419) -> (-46.125, 25.3701)
  line L855 (-45.8779, 25.0789) -> (-45.4869, 25.4023)
  line L856 (-45.4869, 25.4023) -> (-45.1173, 25.7505)
  line L857 (-45.1173, 25.7505) -> (-45.5094, 25.4281)
  line L858 (-45.5094, 25.4281) -> (-45.8779, 25.0789)
  line L859 (-45.677, 24.922) -> (-45.2419, 25.268)
  line L860 (-45.2419, 25.268) -> (-44.8272, 25.6387)
  line L861 (-44.8272, 25.6387) -> (-45.2623, 25.2938)
  line L862 (-45.2623, 25.2938) -> (-45.677, 24.922)
  line L863 (-45.6545, 24.5652) -> (-45.0958, 25.0327)
  line L864 (-45.0958, 25.0327) -> (-44.5587, 25.527)
  line L865 (-44.5587, 25.527) -> (-45.1173, 25.0585)
  line L866 (-45.1173, 25.0585) -> (-45.6545, 24.5652)
  line L867 (-45.431, 24.3847) -> (-44.9723, 24.7866)
  line L868 (-44.9723, 24.7866) -> (-44.535, 25.2132)
  line L869 (-44.535, 25.2132) -> (-44.9948, 24.8113)
  line L870 (-44.9948, 24.8113) -> (-45.431, 24.3847)
  line L871 (-45.2967, 24.0946) -> (-44.882, 24.4857)
  line L872 (-44.882, 24.4857) -> (-44.491, 24.9005)
  line L873 (-44.491, 24.9005) -> (-44.9057, 24.5093)
  line L874 (-44.9057, 24.5093) -> (-45.2967, 24.0946)
  line L875 (-44.9615, 24.0946) -> (-44.636, 24.3847)
  line L876 (-44.636, 24.3847) -> (-44.3341, 24.6995)
  line L877 (-44.3341, 24.6995) -> (-44.6596, 24.4083)
  line L878 (-44.6596, 24.4083) -> (-44.9615, 24.0946)
  line L879 (-44.8487, 23.7808) -> (-44.5232, 24.116)
  line L880 (-44.5232, 24.116) -> (-44.2224, 24.4749)
  line L881 (-44.2224, 24.4749) -> (-44.5479, 24.1386)
  line L882 (-44.5479, 24.1386) -> (-44.8487, 23.7808)
  line L883 (-44.4459, 23.8033) -> (-44.2095, 24.072)
  line L884 (-44.2095, 24.072) -> (-43.9979, 24.3632)
  line L885 (-43.9979, 24.3632) -> (-44.2353, 24.0935)
  line L886 (-44.2353, 24.0935) -> (-44.4459, 23.8033)
  line L887 (-43.7078, 24.2729) -> (-44, 23.9592)
  line L888 (-44, 23.9592) -> (-44.2665, 23.6239)
  line L889 (-44.2665, 23.6239) -> (-43.9742, 23.9377)
  line L890 (-43.9742, 23.9377) -> (-43.7078, 24.2729)
  line L891 (-43.6627, 23.9602) -> (-43.9893, 23.6239)
  line L892 (-43.9893, 23.6239) -> (-44.2901, 23.266)
  line L893 (-44.2901, 23.266) -> (-43.9635, 23.6013)
  line L894 (-43.9635, 23.6013) -> (-43.6627, 23.9602)
  line L895 (-43.5058, 23.8033) -> (-43.7551, 23.5003)
  line L896 (-43.7551, 23.5003) -> (-43.9764, 23.1758)
  line L897 (-43.9764, 23.1758) -> (-43.7271, 23.4799)
  line L898 (-43.7271, 23.4799) -> (-43.5058, 23.8033)
  line L899 (-43.1707, 23.7582) -> (-43.4865, 23.3542)
  line L900 (-43.4865, 23.3542) -> (-43.7744, 22.9297)
  line L901 (-43.7744, 22.9297) -> (-43.4586, 23.3337)
  line L902 (-43.4586, 23.3337) -> (-43.1707, 23.7582)
  line L903 (-42.9687, 23.7808) -> (-43.3307, 23.1844)
  line L904 (-43.3307, 23.1844) -> (-43.6627, 22.5718)
  line L905 (-43.6627, 22.5718) -> (-43.3017, 23.1682)
  line L906 (-43.3017, 23.1682) -> (-42.9687, 23.7808)
  line L907 (-43.2373, 22.7062) -> (-43.0546, 22.977)
  line L908 (-43.0546, 22.977) -> (-42.9021, 23.266)
  line L909 (-42.9021, 23.266) -> (-43.0847, 22.9952)
  line L910 (-43.0847, 22.9952) -> (-43.2373, 22.7062)
  line L911 (-41.8278, 22.617) -> (-42.033, 22.2441)
  line L912 (-42.033, 22.2441) -> (-42.2081, 21.8551)
  line L913 (-42.2081, 21.8551) -> (-42.0029, 22.2291)
  line L914 (-42.0029, 22.2291) -> (-41.8278, 22.617)
  line L915 (-41.5807, 22.5718) -> (-41.7988, 22.0636)
  line L916 (-41.7988, 22.0636) -> (-41.9836, 21.5424)
  line L917 (-41.9836, 21.5424) -> (-41.7665, 22.0507)
  line L918 (-41.7665, 22.0507) -> (-41.5807, 22.5718)
  line L919 (-41.6258, 21.8551) -> (-41.7204, 21.6488)
  line L920 (-41.7204, 21.6488) -> (-41.7827, 21.4296)
  line L921 (-41.7827, 21.4296) -> (-41.6892, 21.637)
  line L922 (-41.6892, 21.637) -> (-41.6258, 21.8551)
  line L923 (-41.0435, 22.3698) -> (-41.3175, 21.7272)
  line L924 (-41.3175, 21.7272) -> (-41.5592, 21.0717)
  line L925 (-41.5592, 21.0717) -> (-41.2863, 21.7154)
  line L926 (-41.2863, 21.7154) -> (-41.0435, 22.3698)
  line L927 (-40.8201, 22.2581) -> (-40.9049, 21.4768)
  line L928 (-40.9049, 21.4768) -> (-40.9544, 20.6913)
  line L929 (-40.9544, 20.6913) -> (-40.8706, 21.4736)
  line L930 (-40.8706, 21.4736) -> (-40.8201, 22.2581)
  spline S2165 degree 3 poles (-40.0369, 21.2512) (-40.0369, 21.0287) (-40.009, 20.744) (-39.9649, 20.514) knots 0 0 0 0 1 1 1 1
  spline S2166 degree 3 poles (-39.9649, 20.514) (-39.9198, 20.284) (-39.8521, 20.1142) (-39.851, 20.111) knots 0 0 0 0 1 1 1 1
  line L931 (-39.851, 20.111) -> (-39.9316, 20.5194)
  spline S2167 degree 3 poles (-39.9316, 20.5194) (-39.9757, 20.7483) (-40.0369, 21.0309) (-40.0369, 21.2512) knots 0 0 0 0 1 1 1 1
  spline S2168 degree 3 poles (-39.59, 20.7364) (-39.5775, 20.5294) (-39.5426, 20.3244) (-39.4858, 20.125) knots 0 0 0 0 1 1 1 1
  spline S2169 degree 3 poles (-39.4858, 20.125) (-39.4331, 19.9455) (-39.3601, 19.8241) (-39.359, 19.8209) knots 0 0 0 0 1 1 1 1
  line L932 (-39.359, 19.8209) -> (-39.4536, 20.1347)
  spline S2170 degree 3 poles (-39.4536, 20.1347) (-39.5073, 20.312) (-39.5782, 20.5387) (-39.59, 20.7364) knots 0 0 0 0 1 1 1 1
  line L933 (-39.214, 20.2045) -> (-39.0743, 19.8402)
  line L934 (-39.0743, 19.8402) -> (-39.1818, 20.2153)
  line L935 (-39.1818, 20.2153) -> (-39.3214, 20.5806)
  line L936 (-39.3214, 20.5806) -> (-39.214, 20.2045)
  spline S2171 degree 3 poles (-39.2763, 21.2512) (-39.2763, 21.2458) (-39.2924, 21.1824) (-39.272, 21.0674) knots 0 0 0 0 1 1 1 1
  spline S2172 degree 3 poles (-39.272, 21.0674) (-39.2348, 20.9012) (-39.1838, 20.7383) (-39.1195, 20.5806) knots 0 0 0 0 1 1 1 1
  spline S2173 degree 3 poles (-39.1195, 20.5806) (-39.1968, 20.788) (-39.2194, 20.9589) (-39.2398, 21.0739) knots 0 0 0 0 1 1 1 1
  spline S2174 degree 3 poles (-39.2398, 21.0739) (-39.2591, 21.1878) (-39.2763, 21.2501) (-39.2763, 21.2512) knots 0 0 0 0 1 1 1 1
  spline S2175 degree 3 poles (-38.94, 20.8482) (-38.9368, 20.8364) (-38.9196, 20.6913) (-38.8691, 20.5312) knots 0 0 0 0 1 1 1 1
  spline S2176 degree 3 poles (-38.8691, 20.5312) (-38.8186, 20.37) (-38.7391, 20.1991) (-38.6715, 20.1089) knots 0 0 0 0 1 1 1 1
  spline S2177 degree 3 poles (-38.6715, 20.1089) (-38.737, 20.1959) (-38.7896, 20.3883) (-38.8401, 20.5495) knots 0 0 0 0 1 1 1 1
  spline S2178 degree 3 poles (-38.8401, 20.5495) (-38.8906, 20.7096) (-38.939, 20.846) (-38.94, 20.8482) knots 0 0 0 0 1 1 1 1
  spline S2179 degree 3 poles (-38.7391, 20.9374) (-38.737, 20.932) (-38.6392, 20.673) (-38.5028, 20.3797) knots 0 0 0 0 1 1 1 1
  spline S2180 degree 3 poles (-38.5028, 20.3797) (-38.377, 20.1117) (-38.239, 19.8495) (-38.0892, 19.5941) knots 0 0 0 0 1 1 1 1
  spline S2181 degree 3 poles (-38.0892, 19.5941) (-38.1891, 19.7596) (-38.3363, 20.1014) (-38.4727, 20.3947) knots 0 0 0 0 1 1 1 1
  spline S2182 degree 3 poles (-38.4727, 20.3947) (-38.6092, 20.687) (-38.737, 20.932) (-38.7391, 20.9374) knots 0 0 0 0 1 1 1 1
  spline S2183 degree 3 poles (-38.4254, 20.8256) (-38.4147, 20.7998) (-38.3008, 20.4785) (-38.1493, 20.1433) knots 0 0 0 0 1 1 1 1
  spline S2184 degree 3 poles (-38.1493, 20.1433) (-37.9968, 19.8069) (-37.8099, 19.4598) (-37.71, 19.3481) knots 0 0 0 0 1 1 1 1
  spline S2185 degree 3 poles (-37.71, 19.3481) (-37.8088, 19.4577) (-37.9732, 19.8338) (-38.1257, 20.1734) knots 0 0 0 0 1 1 1 1
  spline S2186 degree 3 poles (-38.1257, 20.1734) (-38.2783, 20.5119) (-38.4233, 20.8192) (-38.4254, 20.8256) knots 0 0 0 0 1 1 1 1
  spline S2187 degree 3 poles (-38.4469, 21.3855) (-38.4448, 21.379) (-38.2955, 21.0212) (-38.058, 20.5688) knots 0 0 0 0 1 1 1 1
  spline S2188 degree 3 poles (-38.058, 20.5688) (-37.8195, 20.1153) (-37.494, 19.5684) (-37.1932, 19.146) knots 0 0 0 0 1 1 1 1
  spline S2189 degree 3 poles (-37.1932, 19.146) (-37.4919, 19.5662) (-37.7895, 20.1314) (-38.0269, 20.5839) knots 0 0 0 0 1 1 1 1
  spline S2190 degree 3 poles (-38.0269, 20.5839) (-38.2654, 21.0362) (-38.4448, 21.379) (-38.4469, 21.3855) knots 0 0 0 0 1 1 1 1
  spline S2191 degree 3 poles (-37.9785, 21.0051) (-37.9753, 20.9986) (-37.8485, 20.7149) (-37.6412, 20.3431) knots 0 0 0 0 1 1 1 1
  spline S2192 degree 3 poles (-37.6412, 20.3431) (-37.4339, 19.9702) (-37.147, 19.5125) (-36.8806, 19.1245) knots 0 0 0 0 1 1 1 1
  spline S2193 degree 3 poles (-36.8806, 19.1245) (-37.147, 19.5114) (-37.4059, 19.9874) (-37.6133, 20.3593) knots 0 0 0 0 1 1 1 1
  spline S2194 degree 3 poles (-37.6133, 20.3593) (-37.8185, 20.7311) (-37.9753, 20.9986) (-37.9785, 21.0051) knots 0 0 0 0 1 1 1 1
  spline S2195 degree 3 poles (-38.0677, 21.6541) (-38.0656, 21.6488) (-37.9581, 21.3457) (-37.6519, 20.8536) knots 0 0 0 0 1 1 1 1
  spline S2196 degree 3 poles (-37.6519, 20.8536) (-37.3447, 20.3625) (-36.8398, 19.6876) (-36.0985, 18.9) knots 0 0 0 0 1 1 1 1
  spline S2197 degree 3 poles (-36.0985, 18.9) (-36.6708, 19.504) (-37.1811, 20.1639) (-37.6219, 20.8697) knots 0 0 0 0 1 1 1 1
  spline S2198 degree 3 poles (-37.6219, 20.8697) (-37.928, 21.3597) (-38.0656, 21.6488) (-38.0677, 21.6541) knots 0 0 0 0 1 1 1 1
  spline S2199 degree 3 poles (-36.9161, 20.4098) (-37.3608, 20.9632) (-37.5929, 21.3554) (-37.5972, 21.3629) knots 0 0 0 0 1 1 1 1
  spline S2200 degree 3 poles (-37.5972, 21.3629) (-37.5929, 21.3554) (-37.3898, 20.9449) (-36.9418, 20.3904) knots 0 0 0 0 1 1 1 1
  spline S2201 degree 3 poles (-36.9418, 20.3904) (-36.3536, 19.6693) (-35.6621, 19.0389) (-34.8899, 18.5195) knots 0 0 0 0 1 1 1 1
  spline S2202 degree 3 poles (-34.8899, 18.5195) (-35.6549, 19.046) (-36.3377, 19.683) (-36.9161, 20.4098) knots 0 0 0 0 1 1 1 1
  spline S2203 degree 3 poles (-37.3737, 21.4296) (-37.3662, 21.4199) (-36.9698, 20.9084) (-36.3445, 20.2894) knots 0 0 0 0 1 1 1 1
  spline S2204 degree 3 poles (-36.3445, 20.2894) (-35.7193, 19.6715) (-34.8695, 18.9515) (-33.9939, 18.4755) knots 0 0 0 0 1 1 1 1
  spline S2205 degree 3 poles (-33.9939, 18.4755) (-34.8663, 18.9505) (-35.6978, 19.6984) (-36.322, 20.3141) knots 0 0 0 0 1 1 1 1
  spline S2206 degree 3 poles (-36.322, 20.3141) (-36.945, 20.9309) (-37.3662, 21.4199) (-37.3737, 21.4296) knots 0 0 0 0 1 1 1 1
  spline S2207 degree 3 poles (-36.6357, 21.0491) (-36.626, 21.0405) (-36.1576, 20.5828) (-35.5044, 20.0487) knots 0 0 0 0 1 1 1 1
  spline S2208 degree 3 poles (-35.5044, 20.0487) (-34.8523, 19.5146) (-34.0208, 18.9075) (-33.345, 18.5195) knots 0 0 0 0 1 1 1 1
  spline S2209 degree 3 poles (-33.345, 18.5195) (-34.0186, 18.9064) (-34.8222, 19.5555) (-35.4732, 20.0885) knots 0 0 0 0 1 1 1 1
  spline S2210 degree 3 poles (-35.4732, 20.0885) (-36.1243, 20.6215) (-36.626, 21.0405) (-36.6357, 21.0491) knots 0 0 0 0 1 1 1 1
  spline S2211 degree 3 poles (-36.568, 21.4081) (-36.5551, 21.3973) (-35.9331, 20.8256) (-35.1048, 20.2024) knots 0 0 0 0 1 1 1 1
  spline S2212 degree 3 poles (-35.1048, 20.2024) (-34.2765, 19.5791) (-33.2484, 18.9086) (-32.4931, 18.5872) knots 0 0 0 0 1 1 1 1
  spline S2213 degree 3 poles (-32.4931, 18.5872) (-33.2441, 18.9064) (-34.24, 19.6361) (-35.0672, 20.2572) knots 0 0 0 0 1 1 1 1
  spline S2214 degree 3 poles (-35.0672, 20.2572) (-35.571, 20.6361) (-36.0713, 21.0198) (-36.568, 21.4081) knots 0 0 0 0 1 1 1 1
  spline S2215 degree 3 poles (-36.1651, 21.5424) (-36.1501, 21.5306) (-35.4152, 20.9417) (-34.4784, 20.3045) knots 0 0 0 0 1 1 1 1
  spline S2216 degree 3 poles (-34.4784, 20.3045) (-33.5417, 19.6683) (-32.4094, 18.987) (-31.6659, 18.6764) knots 0 0 0 0 1 1 1 1
  spline S2217 degree 3 poles (-31.6659, 18.6764) (-32.405, 18.9849) (-33.5083, 19.7263) (-34.443, 20.3614) knots 0 0 0 0 1 1 1 1
  spline S2218 degree 3 poles (-34.443, 20.3614) (-35.3766, 20.9976) (-36.1501, 21.5306) (-36.1651, 21.5424) knots 0 0 0 0 1 1 1 1
  spline S2219 degree 3 poles (-35.1585, 21.2952) (-35.1434, 21.2866) (-34.4086, 20.7988) (-33.5126, 20.2604) knots 0 0 0 0 1 1 1 1
  spline S2220 degree 3 poles (-33.5126, 20.2604) (-32.6761, 19.7539) (-31.8215, 19.2779) (-30.9505, 18.8333) knots 0 0 0 0 1 1 1 1
  spline S2221 degree 3 poles (-30.9505, 18.8333) (-31.5585, 19.1321) (-32.5908, 19.765) (-33.4869, 20.3034) knots 0 0 0 0 1 1 1 1
  spline S2222 degree 3 poles (-33.4869, 20.3034) (-34.3817, 20.8417) (-35.1434, 21.2866) (-35.1585, 21.2952) knots 0 0 0 0 1 1 1 1
  line L937 (-34.6879, 21.4296) -> (-32.4244, 20.139)
  line L938 (-32.4244, 20.139) -> (-30.1447, 18.8785)
  line L939 (-30.1447, 18.8785) -> (-32.4072, 20.1691)
  line L940 (-32.4072, 20.1691) -> (-34.6879, 21.4296)
  spline S2223 degree 3 poles (-31.8689, 20.4345) (-32.6769, 20.8869) (-33.4224, 21.2608) (-33.4364, 21.2673) knots 0 0 0 0 1 1 1 1
  spline S2224 degree 3 poles (-33.4364, 21.2673) (-33.4224, 21.2598) (-32.6929, 20.8579) (-31.8883, 20.4065) knots 0 0 0 0 1 1 1 1
  spline S2225 degree 3 poles (-31.8883, 20.4065) (-31.0826, 19.9541) (-30.1963, 19.4566) (-29.8965, 19.2137) knots 0 0 0 0 1 1 1 1
  spline S2226 degree 3 poles (-29.8965, 19.2137) (-30.1974, 19.4577) (-31.0632, 19.9821) (-31.8689, 20.4345) knots 0 0 0 0 1 1 1 1
  spline S2227 degree 3 poles (-33.6835, 21.8272) (-33.6684, 21.8196) (-32.8895, 21.4489) (-31.9152, 20.9374) knots 0 0 0 0 1 1 1 1
  spline S2228 degree 3 poles (-31.9152, 20.9374) (-30.9408, 20.4259) (-29.7644, 19.7768) (-28.9802, 19.1686) knots 0 0 0 0 1 1 1 1
  spline S2229 degree 3 poles (-28.9802, 19.1686) (-29.7655, 19.7779) (-30.9247, 20.4549) (-31.9002, 20.9664) knots 0 0 0 0 1 1 1 1
  spline S2230 degree 3 poles (-31.9002, 20.9664) (-32.8756, 21.479) (-33.6684, 21.8196) (-33.6835, 21.8272) knots 0 0 0 0 1 1 1 1
  spline S2231 degree 3 poles (-33.2108, 22.012) (-33.1903, 22.0034) (-32.1677, 21.5424) (-30.7849, 21.0857) knots 0 0 0 0 1 1 1 1
  spline S2232 degree 3 poles (-30.7849, 21.0857) (-29.4013, 20.6279) (-27.6695, 20.1755) (-26.2504, 20.0863) knots 0 0 0 0 1 1 1 1
  spline S2233 degree 3 poles (-26.2504, 20.0863) (-27.6631, 20.1755) (-29.3905, 20.6773) (-30.77, 21.134) knots 0 0 0 0 1 1 1 1
  spline S2234 degree 3 poles (-30.77, 21.134) (-32.1494, 21.5897) (-33.1904, 22.0034) (-33.2108, 22.012) knots 0 0 0 0 1 1 1 1
  spline S2235 degree 3 poles (-32.1591, 21.9002) (-32.1375, 21.8938) (-31.1642, 21.5563) (-30.0329, 21.2243) knots 0 0 0 0 1 1 1 1
  spline S2236 degree 3 poles (-30.0329, 21.2243) (-28.9027, 20.8923) (-27.6212, 20.5677) (-27.0121, 20.4893) knots 0 0 0 0 1 1 1 1
  spline S2237 degree 3 poles (-27.0121, 20.4893) (-27.619, 20.5677) (-28.8921, 20.9417) (-30.0211, 21.2727) knots 0 0 0 0 1 1 1 1
  line L941 (-30.0211, 21.2727) -> (-32.1591, 21.9002)
  line L942 (-30.4573, 21.6316) -> (-28.8265, 21.2232)
  line L943 (-28.8265, 21.2232) -> (-27.1904, 20.8482)
  line L944 (-27.1904, 20.8482) -> (-28.8201, 21.2565)
  line L945 (-28.8201, 21.2565) -> (-30.4573, 21.6316)
  line L946 (-31.3758, 22.0732) -> (-29.1359, 21.5832)
  spline S2238 degree 3 poles (-29.1359, 21.5832) (-27.9972, 21.3328) (-26.7939, 21.0706) (-26.5393, 20.96) knots 0 0 0 0 1 1 1 1
  spline S2239 degree 3 poles (-26.5393, 20.96) (-26.795, 21.0706) (-27.9541, 21.3576) (-29.0779, 21.6047) knots 0 0 0 0 1 1 1 1
  spline S2240 degree 3 poles (-29.0779, 21.6047) (-30.2027, 21.8529) (-31.2877, 22.055) (-31.3758, 22.0732) knots 0 0 0 0 1 1 1 1
  spline S2241 degree 3 poles (-31.8916, 22.4988) (-31.8689, 22.4934) (-30.8076, 22.2473) (-29.6323, 21.9711) knots 0 0 0 0 1 1 1 1
  spline S2242 degree 3 poles (-29.6323, 21.9711) (-28.4591, 21.695) (-27.1732, 21.3941) (-26.7198, 21.2286) knots 0 0 0 0 1 1 1 1
  spline S2243 degree 3 poles (-26.7198, 21.2286) (-27.1742, 21.3952) (-28.4505, 21.7272) (-29.6248, 22.0045) knots 0 0 0 0 1 1 1 1
  spline S2244 degree 3 poles (-29.6248, 22.0045) (-30.799, 22.2806) (-31.8689, 22.4934) (-31.8916, 22.4988) knots 0 0 0 0 1 1 1 1
  spline S2245 degree 3 poles (-29.8053, 22.3387) (-28.7299, 22.1216) (-27.5427, 21.8755) (-27.1001, 21.6982) knots 0 0 0 0 1 1 1 1
  spline S2246 degree 3 poles (-27.1001, 21.6982) (-27.5438, 21.8755) (-28.7213, 22.1538) (-29.7976, 22.3709) knots 0 0 0 0 1 1 1 1
  spline S2247 degree 3 poles (-29.7976, 22.3709) (-30.8752, 22.589) (-31.8496, 22.7416) (-31.8689, 22.7449) knots 0 0 0 0 1 1 1 1
  spline S2248 degree 3 poles (-31.8689, 22.7449) (-31.8496, 22.7416) (-30.8816, 22.5568) (-29.8053, 22.3387) knots 0 0 0 0 1 1 1 1
  spline S2249 degree 3 poles (-29.5173, 22.617) (-29.7516, 22.7287) (-30.3455, 22.8641) (-30.8988, 22.9587) knots 0 0 0 0 1 1 1 1
  spline S2250 degree 3 poles (-30.8988, 22.9587) (-31.4533, 23.0522) (-31.9614, 23.0973) (-32.0021, 23.1027) knots 0 0 0 0 1 1 1 1
  spline S2251 degree 3 poles (-32.0021, 23.1027) (-31.9925, 23.1016) (-31.4887, 23.0232) (-30.9289, 22.9286) knots 0 0 0 0 1 1 1 1
  spline S2252 degree 3 poles (-30.9289, 22.9286) (-30.3713, 22.8341) (-29.7494, 22.7266) (-29.5173, 22.617) knots 0 0 0 0 1 1 1 1
  spline S2253 degree 3 poles (-46.7202, 32.7301) (-46.833, 32.4947) (-46.9114, 32.2217) (-46.9887, 31.8048) knots 0 0 0 0 1 1 1 1
  line L947 (-46.9887, 31.8048) -> (-46.9006, 31.7962)
  spline S2254 degree 3 poles (-46.9006, 31.7962) (-46.9006, 31.8134) (-46.8964, 31.8338) (-46.8888, 31.8531) knots 0 0 0 0 1 1 1 1
  spline S2255 degree 3 poles (-46.8888, 31.8531) (-46.8426, 32.2077) (-46.646, 32.5924) (-46.5913, 32.6924) knots 0 0 0 0 1 1 1 1
  line L948 (-46.5913, 32.6924) -> (-46.7202, 32.7301)
  line L949 (-46.429, 31.8735) -> (-46.3656, 32.1024)
  spline S2256 degree 3 poles (-46.3656, 32.1024) (-46.992, 32.2411) (-46.587, 31.9703) (-46.429, 31.8735) knots 0 0 0 0 1 1 1 1
  spline S2257 degree 3 poles (-46.8813, 31.8338) (-46.8833, 31.8155) (-46.8855, 31.7972) (-46.8878, 31.779) knots 0 0 0 0 1 1 1 1
  line L950 (-46.8878, 31.779) -> (-46.4645, 31.7435)
  line L951 (-46.4645, 31.7435) -> (-46.4333, 31.8585)
  spline S2258 degree 3 poles (-46.4333, 31.8585) (-46.7073, 31.938) (-46.8523, 31.9004) (-46.8813, 31.8338) knots 0 0 0 0 1 1 1 1
  line L952 (-46.2786, 32.3937) -> (-46.226, 32.5892)
  line L953 (-46.226, 32.5892) -> (-46.3614, 32.629)
  spline S2259 degree 3 poles (-46.3614, 32.629) (-46.8716, 32.6773) (-46.3656, 32.4356) (-46.2786, 32.3937) knots 0 0 0 0 1 1 1 1
  line L954 (-46.3592, 32.1089) -> (-46.2851, 32.3775)
  spline S2260 degree 3 poles (-46.2851, 32.3775) (-47.0532, 32.5097) (-46.4129, 32.1401) (-46.3592, 32.1089) knots 0 0 0 0 1 1 1 1
  spline S2261 degree 3 poles (-45.9735, 31.2922) (-46.0498, 31.5329) (-46.2797, 31.4244) (-46.2647, 31.275) knots 0 0 0 0 1 1 1 1
  spline S2262 degree 3 poles (-46.2647, 31.275) (-45.2387, 26.4802) (-42.3585, 24.5083) (-40.3947, 23.7077) knots 0 0 0 0 1 1 1 1
  line L955 (-40.3947, 23.7077) -> (-40.4978, 23.7668)
  spline S2263 degree 3 poles (-40.4978, 23.7668) (-41.5642, 24.2569) (-42.5272, 24.9463) (-43.335, 25.7978) knots 0 0 0 0 1 1 1 1
  spline S2264 degree 3 poles (-43.335, 25.7978) (-44.6672, 27.2055) (-45.4987, 29.0538) (-45.9735, 31.2922) knots 0 0 0 0 1 1 1 1
  spline S2265 degree 3 poles (-46.9652, 31.3137) (-46.7847, 30.2262) (-46.0026, 26.9294) (-42.9451, 24.6007) knots 0 0 0 0 1 1 1 1
  spline S2266 degree 3 poles (-42.9451, 24.6007) (-41.4712, 23.4788) (-39.893, 22.7932) (-38.2568, 22.5611) knots 0 0 0 0 1 1 1 1
  spline S2267 degree 3 poles (-38.2568, 22.5611) (-37.0772, 22.3946) (-35.8847, 22.4848) (-34.9608, 22.8072) knots 0 0 0 0 1 1 1 1
  spline S2268 degree 3 poles (-34.9608, 22.8072) (-34.9501, 22.8158) (-34.9372, 22.8244) (-34.9222, 22.8298) knots 0 0 0 0 1 1 1 1
  spline S2269 degree 3 poles (-34.9222, 22.8298) (-34.9082, 22.8341) (-34.8824, 22.9018) (-34.905, 22.9792) knots 0 0 0 0 1 1 1 1
  spline S2270 degree 3 poles (-34.905, 22.9792) (-34.9254, 23.0469) (-34.9598, 23.0619) (-34.9909, 23.063) knots 0 0 0 0 1 1 1 1
  spline S2271 degree 3 poles (-34.9909, 23.063) (-35.8515, 22.7857) (-36.5874, 22.7847) (-37.0601, 22.7847) knots 0 0 0 0 1 1 1 1
  spline S2272 degree 3 poles (-37.0601, 22.7847) (-37.1524, 22.7847) (-37.8744, 22.7932) (-38.8208, 23.0619) knots 0 0 0 0 1 1 1 1
  spline S2273 degree 3 poles (-38.8208, 23.0619) (-39.9159, 23.2715) (-40.9623, 23.6837) (-41.9062, 24.2773) knots 0 0 0 0 1 1 1 1
  spline S2274 degree 3 poles (-41.9062, 24.2773) (-42.9685, 24.9446) (-43.8843, 25.8205) (-44.5985, 26.852) knots 0 0 0 0 1 1 1 1
  spline S2275 degree 3 poles (-44.5985, 26.852) (-45.4665, 28.0942) (-46.0875, 29.5965) (-46.4463, 31.318) knots 0 0 0 0 1 1 1 1
  spline S2276 degree 3 poles (-46.4463, 31.318) (-46.4946, 31.5673) (-46.9748, 31.4771) (-46.9652, 31.3137) knots 0 0 0 0 1 1 1 1
  spline S2277 degree 2 poles (-46.2475, 31.7855) (-46.2711, 31.7059) (-46.2035, 31.6952) knots 0 0 0 1 1 1
  spline S2278 degree 2 poles (-46.2035, 31.6952) (-46.1369, 31.6823) (-44.1225, 31.5383) knots 0 0 0 1 1 1
  line L956 (-44.1225, 31.5383) -> (-46.2475, 31.7855)
  line L957 (-46.226, 31.8961) -> (-44.2117, 31.6608)
  spline S2279 degree 2 poles (-44.2117, 31.6608) (-46.0692, 31.9961) (-46.1809, 31.9961) knots 0 0 0 1 1 1
  spline S2280 degree 3 poles (-46.1809, 31.9961) (-46.2142, 31.9972) (-46.226, 31.9402) (-46.226, 31.8961) knots 0 0 0 0 1 1 1 1
  line L958 (-46.631, 38.4114) -> (-46.631, 38.2501)
  line L959 (-46.631, 38.2501) -> (-47.383, 38.2501)
  line L960 (-47.383, 38.2501) -> (-47.383, 38.5316)
  spline S2281 degree 3 poles (-47.383, 38.5316) (-47.383, 38.7273) (-47.3272, 38.8402) (-47.1553, 38.8402) knots 0 0 0 0 1 1 1 1
  spline S2282 degree 3 poles (-47.1553, 38.8402) (-47.0167, 38.8402) (-46.9673, 38.7585) (-46.9598, 38.6595) knots 0 0 0 0 1 1 1 1
  line L961 (-46.9598, 38.6595) -> (-46.631, 38.8508)
  line L962 (-46.631, 38.8508) -> (-46.631, 38.6595)
  line L963 (-46.631, 38.6595) -> (-46.9469, 38.4876)
  line L964 (-46.9469, 38.4876) -> (-46.9469, 38.4125)
  line L965 (-46.9469, 38.4125) -> (-46.631, 38.4114)
  spline S2283 degree 3 poles (-47.0747, 38.5543) (-47.0747, 38.6252) (-47.0887, 38.6672) (-47.1714, 38.6672) knots 0 0 0 0 1 1 1 1
  spline S2284 degree 3 poles (-47.1714, 38.6672) (-47.2498, 38.6672) (-47.2552, 38.5833) (-47.2552, 38.5221) knots 0 0 0 0 1 1 1 1
  line L966 (-47.2552, 38.5221) -> (-47.2552, 38.4103)
  line L967 (-47.2552, 38.4103) -> (-47.0747, 38.4103)
  line L968 (-47.0747, 38.4103) -> (-47.0747, 38.5543)
sketch "Sketch3" plane through (0, 1, 0) normal (0, 1, 0) x (-1, 0, 0)
  line L0 (106.825, -60) -> (28.175, -60)
  line L1 (25, -56.825) -> (25, -9.175)
  line L2 (28.175, -6) -> (106.825, -6)
  line L3 (110, -9.175) -> (110, -56.825)
  arc A0 (106.825, -60) -> (110, -56.825) centre (106.825, -56.825) ccw
  arc A1 (110, -9.175) -> (106.825, -6) centre (106.825, -9.175) ccw
  arc A2 (28.175, -6) -> (25, -9.175) centre (28.175, -9.175) ccw
  arc A3 (25, -56.825) -> (28.175, -60) centre (28.175, -56.825) ccw
  point P0 (110, -60)
  point P1 (25, -60)
  point P2 (110, -6)
  dimension "d8" = 85
  dimension "d9" = 54
  dimension "d10" = 3.175
  constraint horizontal L0
  constraint vertical L1
  constraint horizontal L2
  constraint vertical L3
  constraint coincident P0 L0
  constraint coincident P0 L3
  constraint tangent L0 A0
  constraint tangent L3 A0
  constraint coincident P2 L2
  constraint coincident P2 L3
  constraint tangent L2 A1
  constraint tangent L3 A1
  constraint equal A0 A1
  constraint tangent L1 A2
  constraint tangent L2 A2
  constraint equal A0 A2
  constraint coincident P1 L0
  constraint coincident P1 L1
  constraint tangent L0 A3
  constraint tangent L1 A3
  constraint equal A0 A3
  measures "d8" distance of P0 P1
  measures "d9" distance of P0 P2
  measures "d10" radius of A0
extrude "Extrude2" add sketch "Sketch3" along normal blind 1 separate body makes body 2
hidden bodies 1
